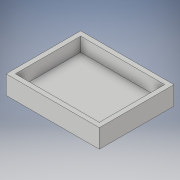
# Autodesk Inventor part: bottom
Saved by Autodesk Inventor 2019 (Build 230136000, 136)
## iProperties
Created: 2021-04-01
Part Number: bottom
Material: Generisch
Document SubType Name: Modeling
Designer: Bergi
Density: 1 g/cm^3
Appearance: Vorgabe
Author: Bergi
Autodesk Inventor part; units mm, degrees
ref_plane "YZ Plane" through (0, 0, 0) normal (1, 0, 0) x (0, 1, 0)
ref_plane "XZ Plane" through (0, 0, 0) normal (0, 1, 0) x (-1, 0, 0)
ref_plane "XY Plane" through (0, 0, 0) normal (0, 0, 1) x (1, 0, 0)
sketch "Skizze1" plane through (0, 0, 0) normal (0, 1, 0) x (-1, 0, 0)
  line L0 (-50, 40) -> (50, 40)
  line L1 (50, 40) -> (50, -40)
  line L2 (50, -40) -> (-50, -40)
  line L3 (-50, -40) -> (-50, 40)
  line L4 (-50, 40) -> (50, -40) construction
  line L5 (50, 40) -> (-50, -40) construction
  point P0 (0, 0)
  dimension "d0" = 100
  dimension "d1" = 80
  constraints: 12 end point, 2 midpoint, 2 parallel, 1 horizontal, 1 perpendicular
  measures "d0" distance of L1.end L2.end
  measures "d1" distance of L0.end L1.end
extrude "Extrusion1" add sketch "Skizze1" along normal blind 5
sketch "Skizze2" plane through (0, 5, 0) normal (0, 1, 0) x (1, 0, 0)
  line L0 (-50, -40) -> (50, -40) projected
  line L1 (50, -40) -> (50, 40) projected
  line L2 (50, 40) -> (-50, 40) projected
  line L3 (-50, 40) -> (-50, -40) projected
  line L4 (-45, -35) -> (45, -35)
  line L5 (45, -35) -> (45, 35)
  line L6 (45, 35) -> (-45, 35)
  line L7 (-45, 35) -> (-45, -35)
  line L8 (-45, -35) -> (45, 35) construction
  line L9 (45, -35) -> (-45, 35) construction
  point P0 (0, 0)
  dimension "d4" = 90
  dimension "d5" = 70
  constraints: 12 end point, 2 midpoint, 2 parallel, 1 horizontal, 1 perpendicular
  measures "d4" distance of L6.end L5.end
  measures "d5" distance of L5.end L4.end
extrude "Extrusion2" add sketch "Skizze2" along normal blind 15
